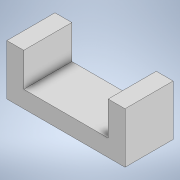
# Autodesk Inventor part: PrintHeadCap
Saved by Autodesk Inventor 2021 (Build 250183000, 183)
## iProperties
Created: 2022-01-21
Part Number: PrintHeadCap
Material: Generic
Document SubType Name: Sheet Metal
Designer: Unit-005
Density: 1 g/cm^3
Sheet Metal Rule: Default
Appearance: Default
Author: Unit-005
Autodesk Inventor part; units mm, degrees
ref_plane "YZ Plane" through (0, 0, 0) normal (1, 0, 0) x (0, 1, 0)
ref_plane "XZ Plane" through (0, 0, 0) normal (0, 1, 0) x (-1, 0, 0)
ref_plane "XY Plane" through (0, 0, 0) normal (0, 0, 1) x (1, 0, 0)
sketch "Sketch1" plane through (0, 0, 0) normal (0, 1, 0) x (-1, 0, 0)
  line L0 (7, -2.85) -> (-7, -2.85)
  line L1 (-7, -2.85) -> (-7, 2.85)
  line L2 (-7, 2.85) -> (7, 2.85)
  line L3 (7, 2.85) -> (7, -2.85)
  line L4 (7, -2.85) -> (-7, 2.85) construction
  line L5 (-7, -2.85) -> (7, 2.85) construction
  point P0 (0, 0)
  dimension "d0" = 14
  dimension "d1" = 5.7
  constraints: 12 end point, 2 midpoint, 2 parallel, 1 horizontal, 1 perpendicular
  measures "d0" distance of L1.end L2.end
  measures "d1" distance of L0.end L1.end
extrude "Extrusion1" add sketch "Sketch1" along normal blind 2
sketch "Sketch2" plane through (0, 2, 0) normal (0, 1, 0) x (1, 0, 0)
  line L0 (7, 2.85) -> (-7, 2.85) projected
  line L1 (-7, -2.85) -> (7, -2.85) projected
  line L2 (-7, 2.85) -> (-5, 2.85)
  line L3 (-5, 2.85) -> (-5, -2.85)
  line L4 (-5, -2.85) -> (-7, -2.85)
  line L5 (-7, -2.85) -> (-7, 2.85)
  line L6 (-9.8, 0) -> (9.8, 0) projected
  line L7 (0, 3.99) -> (0, -3.99) projected
  line L8 (7, 2.85) -> (5, 2.85)
  line L9 (5, 2.85) -> (5, -2.85)
  line L10 (5, -2.85) -> (7, -2.85)
  line L11 (7, -2.85) -> (7, 2.85)
  point P0 (0, 0)
  dimension "d4" = 2
  constraints: 16 end point, 4 symmetric about line, 2 parallel, 1 horizontal, 1 perpendicular, 1 point on line
  measures "d4" distance of L3.end L4.end
extrude "Extrusion2" add sketch "Sketch2" along normal blind 4 contours L11 L6 L9 L0 | L11 L1 L9 L6 | L3 L6 L5 L0 | L3 L1 L5 L6
equation "\"BendRadius\" = Thickness"
equation "\"BendReliefWidth\" = Thickness"
equation "\"BendReliefDepth\" = 0.5 * Thickness"
equation "\"CornerReliefSize\" = 4 * Thickness"
equation "\"MinimumRemnant\" = 2 * Thickness"
equation "\"TransitionRadius\" = BendRadius"
equation "\"JacobiRadiusSize\" = BendRadius"
equation "\"GapSize\" = Thickness"
equation "\"Thickness\" = 3.048"
body "Solid1"
